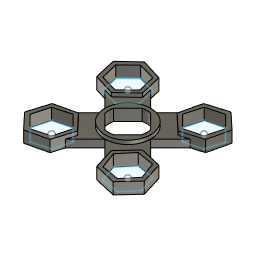
Spinner v1 (Autodesk Fusion 360 design; units mm, degrees)
Autodesk Fusion 360 part; units mm, degrees
sketch "Sketch1" plane through (0, 0, 0) normal (0, 0, 1) x (1, 0, 0)
  circle A0 centre (0, 0) radius 12
  circle A1 centre (0, 0) radius 10
  line L0 (12, 0) -> (0, -12)
  line L1 (-12, 0) -> (0, -12)
  line L2 (-12, 0) -> (0, 12)
  line L3 (0, 12) -> (12, 0)
  line L4 (0, 12) -> (14.1421, 26.1421)
  line L5 (12, 0) -> (26.1421, 14.1421)
  line L6 (26.1421, 14.1421) -> (14.1421, 26.1421)
  line L7 (12, 0) -> (26.1421, -14.1421)
  line L8 (0, -12) -> (14.1421, -26.1421)
  line L9 (14.1421, -26.1421) -> (26.1421, -14.1421)
  line L10 (0, -12) -> (-14.1421, -26.1421)
  line L11 (-12, 0) -> (-26.1421, -14.1421)
  line L12 (-26.1421, -14.1421) -> (-14.1421, -26.1421)
  line L13 (0, 12) -> (-14.1421, 26.1421)
  line L14 (-12, 0) -> (-26.1421, 14.1421)
  line L15 (-26.1421, 14.1421) -> (-14.1421, 26.1421)
  line L16 (16.7761, -9.0966) -> (8.8934, -17.5344)
  line L17 (8.8934, -17.5344) -> (12.2594, -28.5799)
  line L18 (12.2594, -28.5799) -> (23.5081, -31.1876)
  line L19 (23.5081, -31.1876) -> (31.3908, -22.7498)
  line L20 (31.3908, -22.7498) -> (28.0248, -11.7043)
  line L21 (28.0248, -11.7043) -> (16.7761, -9.0966)
  line L22 (-28.0248, -11.7043) -> (-31.3908, -22.7498)
  line L23 (-31.3908, -22.7498) -> (-23.5081, -31.1876)
  line L24 (-23.5081, -31.1876) -> (-12.2594, -28.5799)
  line L25 (-12.2594, -28.5799) -> (-8.8934, -17.5344)
  line L26 (-8.8934, -17.5344) -> (-16.7761, -9.0966)
  line L27 (-16.7761, -9.0966) -> (-28.0248, -11.7043)
  line L28 (-11.7043, 28.0248) -> (-22.7498, 31.3908)
  line L29 (-22.7498, 31.3908) -> (-31.1876, 23.5081)
  line L30 (-31.1876, 23.5081) -> (-28.5799, 12.2594)
  line L31 (-28.5799, 12.2594) -> (-17.5344, 8.8934)
  line L32 (-17.5344, 8.8934) -> (-9.0966, 16.7761)
  line L33 (-9.0966, 16.7761) -> (-11.7043, 28.0248)
  line L34 (9.0966, 16.7761) -> (17.5344, 8.8934)
  line L35 (17.5344, 8.8934) -> (28.5799, 12.2594)
  line L36 (28.5799, 12.2594) -> (31.1876, 23.5081)
  line L37 (31.1876, 23.5081) -> (22.7498, 31.3908)
  line L38 (22.7498, 31.3908) -> (11.7043, 28.0248)
  line L39 (11.7043, 28.0248) -> (9.0966, 16.7761)
  point P0 (20.1421, -20.1421)
  point P1 (-20.1421, -20.1421)
  point P2 (-20.1421, 20.1421)
  point P3 (20.1421, 20.1421)
  dimension "d2" = 20
  dimension "d3" = 20
  dimension "d4" = 20
  dimension "d5" = 20
  dimension "d6" = 20
  dimension "d7" = 20
  dimension "d8" = 20
  dimension "d9" = 20
  dimension "d10" = 10
  dimension "d11" = 10
  dimension "d12" = 10
  dimension "d13" = 10
  constraint coincident A0.centre A1.centre
  constraint coincident A0 L0.start
  constraint coincident A0 L1.start
  constraint coincident A0 L0.end
  constraint perpendicular L0 L1
  constraint coincident A0 L2.end
  constraint perpendicular L1 L2
  constraint perpendicular L3 L4
  constraint perpendicular L3 L5
  constraint perpendicular L5 L7
  constraint perpendicular L0 L8
  constraint perpendicular L1 L10
  constraint perpendicular L1 L11
  constraint perpendicular L2 L13
  constraint perpendicular L2 L14
  constraint midpoint L9 P0
  constraint midpoint L12 P1
  constraint midpoint L15 P2
  constraint midpoint L6 P3
  measures "d2" distance of L2.end L4.end
  measures "d3" distance of L0.start L5.end
  measures "d4" distance of L0.start L7.end
  measures "d5" distance of L0.end L8.end
  measures "d6" distance of L0.end L10.end
  measures "d7" distance of L1.start L11.end
  measures "d8" distance of L2.end L13.end
  measures "d9" distance of L1.start L14.end
  measures "d10" distance of P0 L21
  measures "d11" distance of P1 L27
  measures "d12" distance of P2 L33
  measures "d13" distance of P3 L39
sketch "Sketch2" plane through (0, 0, 0) normal (0, 0, 1) x (1, 0, 0)
  line L0 (-13.3568, 26.4188) -> (-22.2373, 28.9626)
  line L1 (-22.2373, 28.9626) -> (-28.8805, 22.5437)
  line L2 (-28.8805, 22.5437) -> (-26.6432, 13.5812)
  line L3 (-26.6432, 13.5812) -> (-17.7627, 11.0374)
  line L4 (-17.7627, 11.0374) -> (-11.1195, 17.4563)
  line L5 (-11.1195, 17.4563) -> (-13.3568, 26.4188)
  line L6 (17.5255, 11.1) -> (26.4704, 13.407)
  line L7 (26.4704, 13.407) -> (28.9449, 22.307)
  line L8 (28.9449, 22.307) -> (22.4745, 28.9)
  line L9 (22.4745, 28.9) -> (13.5296, 26.593)
  line L10 (13.5296, 26.593) -> (11.0551, 17.693)
  line L11 (11.0551, 17.693) -> (17.5255, 11.1)
  line L12 (10.8946, -18.4429) -> (14.0988, -27.107)
  line L13 (14.0988, -27.107) -> (23.2042, -28.6641)
  line L14 (23.2042, -28.6641) -> (29.1054, -21.5571)
  line L15 (29.1054, -21.5571) -> (25.9012, -12.893)
  line L16 (25.9012, -12.893) -> (16.7958, -11.3359)
  line L17 (16.7958, -11.3359) -> (10.8946, -18.4429)
  line L18 (-17.6342, -11.0705) -> (-26.5503, -13.4864)
  line L19 (-26.5503, -13.4864) -> (-28.9161, -22.4159)
  line L20 (-28.9161, -22.4159) -> (-22.3658, -28.9295)
  line L21 (-22.3658, -28.9295) -> (-13.4497, -26.5136)
  line L22 (-13.4497, -26.5136) -> (-11.0839, -17.5841)
  line L23 (-11.0839, -17.5841) -> (-17.6342, -11.0705)
  point P0 (-20, 20)
  point P1 (20, 20)
  point P2 (20, -20)
  point P3 (-20, -20)
  dimension "d14" = 8
  dimension "d15" = 8
  dimension "d16" = 8
  dimension "d17" = 8
  measures "d14" distance of P0 L5
  measures "d15" distance of P1 L11
  measures "d16" distance of P2 L17
  measures "d17" distance of P3 L23
extrude "Extrude1" add sketch "Sketch2" sketch "Sketch1" along normal blind 6 contours L0 L1 L2 L3 L4 L5 | L6 L7 L8 L9 L10 L11 | L18 L19 L20 L21 L22 L23 of sketch 2 contours L4 L5 L6 L34 L35 L39 | L4 L5 L6 L35 L36 L37 L38 L39 | L7 L8 L9 L17 L18 L19 L20 L21 | L7 L8 L9 L16 L17 L21 | L13 L14 L15 L31 L32 L33 | L13 L14 L15 L28 L29 L30 L31 L33 | L10 L11 L12 L22 L23 L24 L25 L27 | L10 L11 L12 L25 L26 L27 makes body 1 at (23.8917, -21.0114, 0) makes body 2 at (-17.3295, 22.7697, 0) makes body 3 at (23.824, 21.2641, 0) makes body 4 at (-16.3926, -19.2729, 0)
extrude "Extrude2" add sketch "Sketch1" along normal blind 6 separate body contours A0 A1 L3 | A0 A1 L0 | A1 L0 L3 | A0 A1 L2 | A1 L2 L3 | A1 L0 L1 | A0 A1 L1 | A1 L0 | A1 L3 | A1 L1 L2 | A1 L2 | A1 L1 makes body 5
extrude "Extrude3" add sketch "Sketch1" along normal blind 4 contours A0 L7 L8 L16 L17 L21 | A0 L4 L5 L34 L35 L39 | A0 L13 L14 L31 L32 L33 | A0 L10 L11 L25 L26 L27 bodies 5 1 2 3 4
extrude "Extrude4" cut sketch "Sketch2" along normal blind 6 bodies 5
